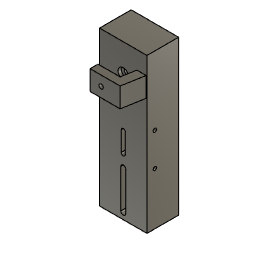
Seitenhalterung für vorne rechts v4 (Autodesk Fusion 360 design; units mm, degrees)
Autodesk Fusion 360 part; units mm, degrees
sketch "Skizze1" plane through (0, 0, 0) normal (0, 0, 1) x (1, 0, 0)
  line L0 (30, 20) -> (-30, 20)
  line L1 (-30, 20) -> (-30, -20)
  line L2 (-30, -20) -> (30, -20)
  line L3 (30, -20) -> (30, 20)
  line L4 (30, 20) -> (-30, -20) construction
  line L5 (-30, 20) -> (30, -20) construction
  dimension "d2" = 60
  dimension "d3" = 40
  constraint perpendicular L0 L1
  constraint parallel L0 L2
  constraint parallel L1 L3
  constraint horizontal L0
  constraint coincident L4 origin
  constraint coincident L5 origin
  measures "d2" distance of L1.end L2.end
  measures "d3" distance of L0.end L1.end
extrude "Extrusion1" add sketch "Skizze1" along normal blind 195 makes body 1
sketch "Skizze3" plane through (0, -20, 0) normal (0, -1, 0) x (1, 0, 0)
  line L0 (-30, 0) -> (30, 0)
  line L1 (30, 0) -> (30, 195)
  line L2 (30, 195) -> (-30, 195)
  line L3 (-30, 195) -> (-30, 0)
  line L4 (3.1, 8.1) -> (3.1, 56.9)
  arc A0 (3.1, 56.9) -> (-3.1, 56.9) centre (0, 56.9) ccw
  line L5 (-3.1, 56.9) -> (-3.1, 8.1)
  arc A1 (-3.1, 8.1) -> (3.1, 8.1) centre (0, 8.1) ccw
  line L6 (0, 5) -> (0, 60) construction
  line L7 (2.5, 72.5) -> (2.5, 97.5)
  arc A2 (2.5, 97.5) -> (-2.5, 97.5) centre (0, 97.5) ccw
  line L8 (-2.5, 97.5) -> (-2.5, 72.5)
  arc A3 (-2.5, 72.5) -> (2.5, 72.5) centre (0, 72.5) ccw
  line L9 (0, 70) -> (0, 100) construction
  point P0 (0, 195)
  dimension "d33" = 6.2
  dimension "d34" = 5
  constraint midpoint L2 P0
  constraint tangent L4 A0
  constraint tangent A0 L5
  constraint parallel L4 L5
  constraint tangent L5 A1
  constraint tangent L4 A1
  constraint midpoint A1 L6.start
  constraint midpoint A0 L6.end
  constraint vertical L6
  constraint tangent L7 A2
  constraint tangent A2 L8
  constraint parallel L7 L8
  constraint tangent L8 A3
  constraint tangent L7 A3
  constraint midpoint A3 L9.start
  constraint midpoint A2 L9.end
  constraint vertical L9
  measures "d33" diameter of A0
  measures "d34" diameter of A2
extrude "Extrusion2" cut sketch "Skizze3" against normal blind 40 contours L4 A0 L5 A1 | L7 A2 L8 A3 bodies 1
sketch "Skizze4" plane through (30, 0, 0) normal (1, 0, 0) x (0, 1, 0)
  line L0 (-20, 0) -> (20, 0)
  line L1 (20, 0) -> (20, 195)
  line L2 (20, 195) -> (-20, 195)
  line L3 (-20, 195) -> (-20, 0)
  circle A0 centre (0, 174.5) radius 4.15
  dimension "d12" = 8.3
  measures "d12" diameter of A0
extrude "Extrusion3" add sketch "Skizze4" against normal blind 60 separate body contours A0 makes body 2
sketch "Skizze6" plane through (0, 0, 0) normal (0, 1, 0) x (1, 0, 0)
sketch "Skizze7" plane through (0, 20, 0) normal (0, 1, 0) x (-1, 0, 0)
  line L0 (-30, 0) -> (30, 0)
  line L1 (30, 0) -> (30, 195)
  line L2 (30, 195) -> (-30, 195)
  line L3 (-30, 195) -> (-30, 0)
  circle A0 centre (0, 160) radius 2.75
  line L4 (-2.5, 72.5) -> (-2.5, 97.5)
  arc A1 (2.5, 97.5) -> (-2.5, 97.5) centre (0, 97.5) ccw
  line L5 (2.5, 97.5) -> (2.5, 72.5)
  arc A2 (-2.5, 72.5) -> (2.5, 72.5) centre (0, 72.5) ccw
  line L6 (-3.1, 8.1) -> (-3.1, 56.9)
  arc A3 (3.1, 56.9) -> (-3.1, 56.9) centre (0, 56.9) ccw
  line L7 (3.1, 56.9) -> (3.1, 8.1)
  arc A4 (-3.1, 8.1) -> (3.1, 8.1) centre (0, 8.1) ccw
  dimension "d17" = 5.5
  measures "d17" diameter of A0
extrude "Extrusion4" cut sketch "Skizze7" against normal blind 40 contours A0 bodies 1
sketch "Skizze9" plane through (30, 0, 0) normal (1, 0, 0) x (0, 1, 0)
  line L0 (-20, 0) -> (20, 0)
  line L1 (20, 0) -> (20, 195)
  line L2 (20, 195) -> (-20, 195)
  line L3 (-20, 195) -> (-20, 0)
  circle A0 centre (-10, 108) radius 2.2
  circle A1 centre (-10, 66) radius 2.2
  dimension "d23" = 4.4
  dimension "d24" = 4.4
  measures "d23" diameter of A0
  measures "d24" diameter of A1
extrude "Extrusion6" cut sketch "Skizze9" against normal blind 80 contours A0 | A1 bodies 1
sketch "Skizze10" plane through (0, 20, 0) normal (0, 1, 0) x (-1, 0, 0)
  circle A0 centre (0, 160) radius 2.75
  line L0 (-30, 0) -> (30, 0)
  line L1 (30, 0) -> (30, 195)
  line L2 (30, 195) -> (-30, 195)
  line L3 (-30, 195) -> (-30, 0)
  circle A1 centre (0, 160) radius 6.65
  line L4 (-2.5, 72.5) -> (-2.5, 97.5)
  arc A2 (2.5, 97.5) -> (-2.5, 97.5) centre (0, 97.5) ccw
  line L5 (2.5, 97.5) -> (2.5, 72.5)
  arc A3 (-2.5, 72.5) -> (2.5, 72.5) centre (0, 72.5) ccw
  line L6 (-3.1, 8.1) -> (-3.1, 56.9)
  arc A4 (3.1, 56.9) -> (-3.1, 56.9) centre (0, 56.9) ccw
  line L7 (3.1, 56.9) -> (3.1, 8.1)
  arc A5 (-3.1, 8.1) -> (3.1, 8.1) centre (0, 8.1) ccw
  dimension "d27" = 13.3
  constraint concentric A0 A1
  measures "d27" diameter of A1
extrude "Extrusion7" cut sketch "Skizze10" against normal blind 4 contours A1 bodies 1
sketch "Skizze11" plane through (0, -20, 0) normal (0, -1, 0) x (1, 0, 0)
  circle A0 centre (0, 160) radius 2.75
  line L0 (-30, 0) -> (30, 0)
  line L1 (30, 0) -> (30, 195)
  line L2 (30, 195) -> (-30, 195)
  line L3 (-30, 195) -> (-30, 0)
  circle A1 centre (0, 160) radius 6.65
  line L4 (2.5, 97.5) -> (2.5, 72.5)
  arc A2 (-2.5, 72.5) -> (2.5, 72.5) centre (0, 72.5) ccw
  line L5 (-2.5, 72.5) -> (-2.5, 97.5)
  arc A3 (2.5, 97.5) -> (-2.5, 97.5) centre (0, 97.5) ccw
  line L6 (3.1, 56.9) -> (3.1, 8.1)
  arc A4 (-3.1, 8.1) -> (3.1, 8.1) centre (0, 8.1) ccw
  line L7 (-3.1, 8.1) -> (-3.1, 56.9)
  arc A5 (3.1, 56.9) -> (-3.1, 56.9) centre (0, 56.9) ccw
  dimension "d30" = 13.3
  constraint concentric A0 A1
  measures "d30" diameter of A1
extrude "Extrusion8" cut sketch "Skizze11" against normal blind 4 contours A1 bodies 1
sketch "Skizze12" plane through (0, 20, 0) normal (0, 1, 0) x (-1, 0, 0)
  circle A0 centre (0, 160) radius 6.65
  line L0 (-2.5, 72.5) -> (-2.5, 97.5)
  arc A1 (2.5, 97.5) -> (-2.5, 97.5) centre (0, 97.5) ccw
  line L1 (2.5, 97.5) -> (2.5, 72.5)
  arc A2 (-2.5, 72.5) -> (2.5, 72.5) centre (0, 72.5) ccw
  line L2 (-3.1, 8.1) -> (-3.1, 56.9)
  arc A3 (3.1, 56.9) -> (-3.1, 56.9) centre (0, 56.9) ccw
  line L3 (3.1, 56.9) -> (3.1, 8.1)
  arc A4 (-3.1, 8.1) -> (3.1, 8.1) centre (0, 8.1) ccw
  line L4 (-30, 0) -> (30, 0)
  line L5 (30, 0) -> (30, 195)
  line L6 (30, 195) -> (-30, 195)
  line L7 (-30, 195) -> (-30, 0)
  line L8 (5, 72.5) -> (5, 97.5)
  arc A5 (5, 97.5) -> (-5, 97.5) centre (0, 97.5) ccw
  line L9 (-5, 97.5) -> (-5, 72.5)
  arc A6 (-5, 72.5) -> (5, 72.5) centre (0, 72.5) ccw
  line L10 (0, 72.5) -> (0, 97.5) construction
  dimension "d35" = 10
  constraint tangent L8 A5
  constraint tangent A5 L9
  constraint parallel L8 L9
  constraint tangent L9 A6
  constraint tangent L8 A6
  constraint coincident A1.centre A5.centre
  constraint parallel L0 L10
  constraint coincident A2.centre A6.centre
  measures "d35" diameter of A5
extrude "Extrusion9" cut sketch "Skizze12" against normal blind 9 contours L8 A5 L9 A6 bodies 1
sketch "Skizze13" plane through (0, -20, 0) normal (0, -1, 0) x (1, 0, 0)
  circle A0 centre (0, 160) radius 6.65
  line L0 (2.5, 97.5) -> (2.5, 72.5)
  arc A1 (-2.5, 72.5) -> (2.5, 72.5) centre (0, 72.5) ccw
  line L1 (-2.5, 72.5) -> (-2.5, 97.5)
  arc A2 (2.5, 97.5) -> (-2.5, 97.5) centre (0, 97.5) ccw
  line L2 (3.1, 56.9) -> (3.1, 8.1)
  arc A3 (-3.1, 8.1) -> (3.1, 8.1) centre (0, 8.1) ccw
  line L3 (-3.1, 8.1) -> (-3.1, 56.9)
  arc A4 (3.1, 56.9) -> (-3.1, 56.9) centre (0, 56.9) ccw
  line L4 (-30, 0) -> (30, 0)
  line L5 (30, 0) -> (30, 195)
  line L6 (30, 195) -> (-30, 195)
  line L7 (-30, 195) -> (-30, 0)
  line L8 (14, 147.5) -> (24, 147.5)
  line L9 (24, 147.5) -> (24, 172.5)
  line L10 (24, 172.5) -> (14, 172.5)
  line L11 (14, 172.5) -> (14, 147.5)
  line L12 (14, 147.5) -> (24, 172.5) construction
  line L13 (24, 147.5) -> (14, 172.5) construction
  point P0 (19, 160)
  dimension "d38" = 25
  dimension "d39" = 10
  constraint perpendicular L8 L9
  constraint parallel L8 L10
  constraint parallel L9 L11
  constraint horizontal L8
  constraint coincident L12 P0
  constraint coincident L13 P0
  measures "d38" distance of L8.end L9.end
  measures "d39" distance of L9.end L10.end
extrude "Extrusion10" add sketch "Skizze13" along normal blind 28 contours L8 L9 L10 L11 bodies 1
sketch "Skizze14" plane through (14, 0, 0) normal (-1, 0, 0) x (0, -1, 0)
  line L0 (20, 172.5) -> (20, 147.5)
  line L1 (20, 147.5) -> (48, 147.5)
  line L2 (48, 147.5) -> (48, 172.5)
  line L3 (48, 172.5) -> (20, 172.5)
  line L4 (48, 172.5) -> (38, 172.5)
  line L5 (38, 172.5) -> (38, 147.5)
  line L6 (38, 147.5) -> (48, 147.5)
  line L7 (48, 147.5) -> (48, 172.5)
  dimension "d42" = 25
  dimension "d43" = 10
  constraint horizontal L4
  constraint vertical L5
  constraint horizontal L6
  constraint vertical L7
  constraint coincident L2.end L3.start
  measures "d42" distance of L2.end L1.end
  measures "d43" distance of L2.end L4.end
extrude "Extrusion11" add sketch "Skizze14" along normal blind 28 contours L1 L2 L3 L4 L5 L6 L7 bodies 1
draft "Entwurf1" angle 10 neutral plane through (14, -48, 147.5) pull (0, -1, 0) 1 faces at (24, -29.3333, 155.8333) on bodies 1
draft "Entwurf2" angle 10 neutral plane through (14, -38, 172.5) pull (0, 1, 0) 1 faces at (14, -26, 164.1667) on bodies 1
sketch "Skizze15" plane through (0, -48, 0) normal (0, -1, 0) x (1, 0, 0)
  line L0 (-14, 147.5) -> (24, 147.5)
  line L1 (24, 147.5) -> (24, 172.5)
  line L2 (24, 172.5) -> (-14, 172.5)
  line L3 (-14, 172.5) -> (-14, 147.5)
  circle A0 centre (0, 160) radius 2.75
  dimension "d50" = 5.5
  measures "d50" diameter of A0
extrude "Extrusion12" cut sketch "Skizze15" against normal blind 10 contours A0 bodies 1
sketch "Skizze16" plane through (0, -38, 0) normal (0, 1, 0) x (-1, 0, 0)
  circle A0 centre (0, 160) radius 2.75
  line L0 (-14, 172.5) -> (-14, 147.5)
  line L1 (-14, 147.5) -> (14, 147.5)
  line L2 (14, 147.5) -> (14, 172.5)
  line L3 (14, 172.5) -> (-14, 172.5)
  circle A1 centre (0, 160) radius 6.65
  dimension "d53" = 13.3
  constraint concentric A0 A1
  measures "d53" diameter of A1
extrude "Extrusion13" cut sketch "Skizze16" against normal blind 4 contours A1 bodies 1
extrude "Extrusion14" cut 1 faces at (-30, -1.0141, 173.1467) along direction (1, 0, 0) blind 50 on bodies 2 bodies 1 2
combine "Kombinieren1" operation add target body 1 tool bodies 2
